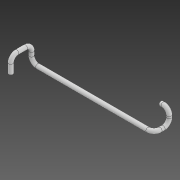
# Autodesk Inventor part: CH_01_0037_syringe_pump_hose
Saved by Autodesk Inventor 2022 (Build 260153000, 153)
## iProperties
Created: 2022-04-22
Part Number: CH_01_0037_syringe_pump_hose
Material: Generic
Document SubType Name: Modeling
Designer: Tomasz Krakowski
Density: 1 g/cm^3
Appearance: Default
Author: Tomasz Krakowski
Autodesk Inventor part; units mm, degrees
ref_plane "YZ Plane" through (0, 0, 0) normal (1, 0, 0) x (0, 1, 0)
ref_plane "XZ Plane" through (0, 0, 0) normal (0, 1, 0) x (-1, 0, 0)
ref_plane "XY Plane" through (0, 0, 0) normal (0, 0, 1) x (1, 0, 0)
sketch "Sketch1" plane through (0, 0, 0) normal (1, 0, 0) x (0, 1, 0)
  circle A0 centre (0, 0) radius 2
  circle A1 centre (0, 0) radius 1
  dimension "d0" = 4
  dimension "d1" = 2
  constraints: 2 centre point, 2 coincident
  measures "d0" diameter of A0
  measures "d1" diameter of A1
sketch3d "3D Sketch1"
  line L0 (0, 0, 0) -> (2, 0, 0)
  arc A0 (2, 0, 0) -> (8, -6, 0) centre (2, -6, 0) ccw
  line L1 (8, -6, 0) -> (8, -8, 0)
  arc A1 (8, -8, 0) -> (8, -14, 6) centre (8, -8, 6) ccw
  line L2 (8, -14, 6) -> (8, -14, 9)
  arc A2 (8, -14, 9) -> (2, -14, 15) centre (2, -14, 9) ccw
  line L3 (2, -14, 15) -> (-106.45, -14, 15)
  arc A3 (-106.45, -14, 15) -> (-112.45, -8, 15) centre (-106.45, -8, 15) ccw
  line L4 (-112.45, -8, 15) -> (-112.45, -4, 15)
  arc A4 (-112.45, -4, 15) -> (-112.45, 2, 21) centre (-112.45, -4, 21) ccw
  line L5 (-112.45, 2, 21) -> (-112.45, 2, 29.4)
  arc A5 (-112.45, 2, 29.4) -> (-112.45, -4, 35.4) centre (-112.45, -4, 29.4) ccw
  line L6 (-112.45, -4, 35.4) -> (-112.45, -13, 35.4)
  dimension "d2" = 14
  dimension "d3" = 8
  dimension "d4" = 15
  dimension "d5" = 120.45
  dimension "d6" = 6
  dimension "d7" = 6
  dimension "d8" = 6
  dimension "d11" = 16
  dimension "d12" = 20.4
  dimension "d13" = 15
  dimension "d14" = 6
  dimension "d15" = 6
  dimension "d16" = 6
sweep "Sweep1" add profiles "Sketch1" path "3D Sketch1"
equation "\"d7\" = d6"
equation "\"d8\" = d6"
equation "\"d15\" = d14"
equation "\"d16\" = d14"
body "Solid1"
